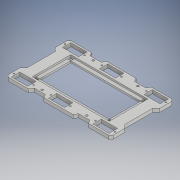
# Autodesk Inventor part: BODY_TOP
Saved by Autodesk Inventor 2017 (Build 210142000, 142)
## iProperties
Created: 2017-09-24
Part Number: BODY_TOP
Material: Generic
Document SubType Name: Modeling
Designer: Alexander Miller
Density: 1 g/cm^3
Appearance: Default
body_C_Top: 5,000 mm
Author: Alexander Miller
Autodesk Inventor part; units mm, degrees
ref_plane "YZ Plane" through (0, 0, 0) normal (1, 0, 0) x (0, 1, 0)
ref_plane "XZ Plane" through (0, 0, 0) normal (0, 1, 0) x (-1, 0, 0)
ref_plane "XY Plane" through (0, 0, 0) normal (0, 0, 1) x (1, 0, 0)
sketch "Sketch1" plane through (0, 0, 0) normal (0, 1, 0) x (-1, 0, 0)
  line L0 (45, -75) -> (-45, -75)
  line L1 (-45, -75) -> (-45, 75)
  line L2 (-45, 75) -> (45, 75)
  line L3 (45, 75) -> (45, -75)
  point P0 (0, 0)
  point P1 (0, -75)
  point P2 (45, 0)
  dimension "d0" = 90
  dimension "d1" = 150
  constraints: 8 end point, 2 midpoint, 2 parallel, 1 horizontal, 1 horizontal alignment, 1 perpendicular, 1 vertical alignment
  measures "d0" distance of L0.start L0.end
  measures "d1" distance of L2.end L0.start
extrude "Extrusion1" add sketch "Sketch1" along normal blind 5
sketch "Sketch2" plane through (0, 5, 0) normal (0, 1, 0) x (1, 0, 0)
  line L0 (-42.5, 69.75) -> (-30.5, 69.75)
  line L1 (-30.5, 69.75) -> (-30.5, 46.75)
  line L2 (-30.5, 46.75) -> (-42.5, 46.75)
  line L3 (-42.5, 46.75) -> (-42.5, 69.75)
  line L4 (-42.5, 17) -> (-30.5, 17)
  line L5 (-30.5, 17) -> (-30.5, -6)
  line L6 (-30.5, -6) -> (-42.5, -6)
  line L7 (-42.5, -6) -> (-42.5, 17)
  line L8 (-42.5, -46.75) -> (-30.5, -46.75)
  line L9 (-30.5, -46.75) -> (-30.5, -69.75)
  line L10 (-30.5, -69.75) -> (-42.5, -69.75)
  line L11 (-42.5, -69.75) -> (-42.5, -46.75)
  line L12 (-45, 75) -> (-45, -75) projected
  line L13 (45, 75) -> (-45, 75) projected
  line L14 (-45, -75) -> (45, -75) projected
  circle A0 centre (-36.5, 0) radius 6 construction
  circle A1 centre (-36.5, 72.25) radius 1
  circle A2 centre (-36.5, 44.25) radius 1
  circle A3 centre (-36.5, 19.5) radius 1
  circle A4 centre (-36.5, -8.5) radius 1
  circle A5 centre (-36.5, -44.25) radius 1
  circle A6 centre (-36.5, -72.25) radius 1
  line L15 (0, 105) -> (0, -105) construction
  line L16 (42.5, 69.75) -> (30.5, 69.75)
  line L17 (30.5, 69.75) -> (30.5, 46.75)
  line L18 (30.5, 46.75) -> (42.5, 46.75)
  line L19 (42.5, 46.75) -> (42.5, 69.75)
  line L20 (42.5, 17) -> (30.5, 17)
  line L21 (30.5, 17) -> (30.5, -6)
  line L22 (30.5, -6) -> (42.5, -6)
  line L23 (42.5, -6) -> (42.5, 17)
  line L24 (42.5, -46.75) -> (30.5, -46.75)
  line L25 (30.5, -46.75) -> (30.5, -69.75)
  line L26 (30.5, -69.75) -> (42.5, -69.75)
  line L27 (42.5, -69.75) -> (42.5, -46.75)
  circle A7 centre (36.5, 72.25) radius 1
  circle A8 centre (36.5, 44.25) radius 1
  circle A9 centre (36.5, 19.5) radius 1
  circle A10 centre (36.5, -8.5) radius 1
  circle A11 centre (36.5, -44.25) radius 1
  circle A12 centre (36.5, -72.25) radius 1
  point P0 (0, 0)
  point P1 (-36.5, 46.75)
  point P2 (-36.5, 17)
  point P3 (-36.5, -6)
  point P4 (-36.5, -46.75)
  point P5 (-36.5, 69.75)
  point P6 (-36.5, -69.75)
  dimension "d2" = 5
  dimension "d4" = 2.5
  dimension "d5" = 5.25
  dimension "d6" = 23
  dimension "d7" = 12
  dimension "d8" = 5.25
  dimension "d9" = 2
  dimension "d10" = 1.5
  dimension "d11" = 1.5
  dimension "d12" = 1.5
  dimension "d13" = 1.5
  dimension "d14" = 1.5
  dimension "d15" = 1.5
  constraints: 48 end point, 18 symmetric about line, 13 centre point, 8 vertical alignment, 6 midpoint, 6 parallel, 5 equal radius, 3 equal length, 3 horizontal, 3 perpendicular, 3 tangent, 2 point on line, 1 horizontal alignment, 6 other
  measures "d4" distance between parallel lines of L3 L12
  measures "d5" distance between parallel lines of L13 L0
  measures "d6" distance of L2.end L0.start
  measures "d7" distance of L0.start L0.end
  measures "d8" distance between parallel lines of L14 L10
  measures "d9" diameter of A1
  measures "d10" distance edge to line of A1 L0
  measures "d11" distance edge to line of A2 L2
  measures "d12" distance edge to line of A3 L4
  measures "d13" distance edge to line of A4 L6
  measures "d14" distance edge to line of A5 L8
  measures "d15" distance edge to line of A6 L10
extrude "Extrusion2" cut sketch "Sketch2" against normal through all
sketch "Sketch3" plane through (0, 5, 0) normal (0, 1, 0) x (1, 0, 0)
  line L0 (45, 42.875) -> (40, 39.875)
  line L1 (40, 39.875) -> (40, 23.875)
  line L2 (45, -75) -> (45, 75) projected
  line L3 (40, 23.875) -> (45, 20.875)
  line L4 (45, 20.875) -> (45, 42.875)
  line L5 (42.5, 46.75) -> (30.5, 46.75) projected
  line L6 (36.5, 46.75) -> (36.5, 17) construction
  line L7 (30.5, 17) -> (42.5, 17) projected
  line L8 (-63, 0) -> (63, 0) projected
  line L9 (0, 105) -> (0, -105) projected
  line L10 (45, -42.875) -> (40, -39.875)
  line L11 (40, -39.875) -> (40, -23.875)
  line L12 (40, -23.875) -> (45, -20.875)
  line L13 (45, -20.875) -> (45, -42.875)
  line L14 (-45, 42.875) -> (-40, 39.875)
  line L15 (-40, 39.875) -> (-40, 23.875)
  line L16 (-40, 23.875) -> (-45, 20.875)
  line L17 (-45, 20.875) -> (-45, 42.875)
  line L18 (-45, -42.875) -> (-40, -39.875)
  line L19 (-40, -39.875) -> (-40, -23.875)
  line L20 (-40, -23.875) -> (-45, -20.875)
  line L21 (-45, -20.875) -> (-45, -42.875)
  line L22 (25, 75) -> (-25, 75)
  line L23 (-25, 75) -> (-20, 70)
  line L24 (-20, 70) -> (20, 70)
  line L25 (20, 70) -> (25, 75)
  line L26 (45, 75) -> (-45, 75) projected
  line L27 (25, -75) -> (-25, -75)
  line L28 (-25, -75) -> (-20, -70)
  line L29 (-20, -70) -> (20, -70)
  line L30 (20, -70) -> (25, -75)
  point P0 (0, 0)
  point P1 (45, 31.875)
  point P2 (40, 31.875)
  point P3 (36.5, 31.875)
  point P4 (0, 70)
  point P5 (0, 75)
  dimension "d38" = 16
  dimension "d39" = 22
  dimension "d40" = 40
  dimension "d41" = 50
  dimension "d42" = 5
  dimension "d43" = 5
  constraints: 50 end point, 16 symmetric about line, 7 midpoint, 3 parallel, 2 collinear, 2 equal length, 2 horizontal alignment, 2 vertical alignment, 1 perpendicular
  measures "d38" distance of L0.end L1.end
  measures "d39" distance of L3.end L0.start
  measures "d40" distance of L23.end L24.end
  measures "d41" distance of L22.start L22.end
  measures "d42" distance between parallel lines of L26 L24
  measures "d43" distance between parallel lines of L1 L4
extrude "Extrusion3" cut sketch "Sketch3" against normal through all contours L2 L3 L1 L0 | L25 L24 L9 L22 | L9 L24 L23 L22 | L10 L11 L12 L2 | L29 L30 L27 L9 | L9 L27 L28 L29 | L14 L15 L16 L17 | L21 L20 L19 L18
chamfer "Chamfer1" distance 3 angle 45 4 edges at (45, 2.5, 75) (-45, 2.5, 75) (-45, 2.5, -75) (45, 2.5, -75)
sketch "Sketch4" plane through (0, 5, 0) normal (0, 1, 0) x (1, 0, 0)
  line L0 (27.5, 55) -> (-27.5, 55)
  line L1 (-27.5, 55) -> (-27.5, -55)
  line L2 (-27.5, -55) -> (27.5, -55)
  line L3 (27.5, -55) -> (27.5, 55)
  line L4 (22.5, 50) -> (-22.5, 50)
  line L5 (-22.5, 50) -> (-22.5, -50)
  line L6 (-22.5, -50) -> (22.5, -50)
  line L7 (22.5, -50) -> (22.5, 50)
  point P0 (0, 0)
  point P1 (27.5, 0)
  point P2 (0, 55)
  dimension "d23" = 110
  dimension "d24" = 55
  dimension "d25" = 5
  dimension "d26" = 5
  dimension "d27" = 5
  dimension "d28" = 5
  constraints: 16 end point, 4 parallel, 2 horizontal, 2 midpoint, 2 perpendicular, 1 horizontal alignment, 1 vertical alignment
  measures "d23" distance of L2.end L0.start
  measures "d24" distance of L1.end L2.end
  measures "d25" distance between parallel lines of L0 L4
  measures "d26" distance between parallel lines of L2 L6
  measures "d27" distance between parallel lines of L3 L7
  measures "d28" distance between parallel lines of L1 L5
extrude "Extrusion4" cut sketch "Sketch4" against normal blind 2.5
sketch "Sketch5" plane through (0, 5, 0) normal (0, 1, 0) x (1, 0, 0)
  line L0 (-22.5, 50) -> (-22.5, -50) projected
  line L1 (-22.5, -50) -> (22.5, -50) projected
  line L2 (22.5, -50) -> (22.5, 50) projected
  line L3 (22.5, 50) -> (-22.5, 50) projected
  point P0 (0, 0)
extrude "Extrusion5" cut sketch "Sketch5" against normal through all
sketch "Sketch6" plane through (0, 2.5, 0) normal (0, 1, 0) x (1, 0, 0)
  line L0 (27.5, 55) -> (22.5, 55)
  line L1 (22.5, 55) -> (22.5, 50)
  line L2 (22.5, 50) -> (27.5, 50)
  line L3 (27.5, 50) -> (27.5, 55)
  line L4 (-63, 0) -> (63, 0) projected
  line L5 (0, 105) -> (0, -105) projected
  line L6 (27.5, -55) -> (22.5, -55)
  line L7 (22.5, -55) -> (22.5, -50)
  line L8 (22.5, -50) -> (27.5, -50)
  line L9 (27.5, -50) -> (27.5, -55)
  line L10 (-27.5, 55) -> (-22.5, 55)
  line L11 (-22.5, 55) -> (-22.5, 50)
  line L12 (-22.5, 50) -> (-27.5, 50)
  line L13 (-27.5, 50) -> (-27.5, 55)
  line L14 (-27.5, -55) -> (-22.5, -55)
  line L15 (-22.5, -55) -> (-22.5, -50)
  line L16 (-22.5, -50) -> (-27.5, -50)
  line L17 (-27.5, -50) -> (-27.5, -55)
  line L18 (27.5, 55) -> (27.5, -55) projected
  line L19 (-27.5, 55) -> (27.5, 55) projected
  point P0 (0, 0)
  dimension "d33" = 5
  dimension "d34" = 5
  constraints: 32 end point, 12 symmetric about line, 2 collinear, 2 parallel, 1 horizontal, 1 perpendicular
  measures "d33" distance of L2.end L0.start
  measures "d34" distance of L1.end L2.end
extrude "Extrusion6" cut sketch "Sketch6" against normal blind 2 contours L3 L2 L1 L0 | L6 L7 L8 L9 | L10 L11 L12 L13 | L17 L16 L15 L14
sketch "Sketch7" plane through (0, 5, 0) normal (0, 1, 0) x (1, 0, 0)
  circle A0 centre (36.5, 31.875) radius 1.5
  line L0 (-63, 0) -> (63, 0) projected
  line L1 (0, 105) -> (0, -105) projected
  line L2 (40, 23.875) -> (40, 39.875) projected
  line L3 (30.5, 17) -> (42.5, 17) projected
  circle A1 centre (36.5, -31.875) radius 1.5
  circle A2 centre (-36.5, 31.875) radius 1.5
  circle A3 centre (-36.5, -31.875) radius 1.5
  point P0 (0, 0)
  point P1 (40, 31.875)
  point P2 (36.5, 17)
  dimension "d44" = 3
  constraints: 4 centre point, 3 symmetric about line, 2 midpoint, 1 horizontal alignment, 1 vertical alignment, 3 other
  measures "d44" diameter of A0
extrude "Extrusion7" cut sketch "Sketch7" against normal through all
sketch "Sketch8" plane through (0, 0, 0) normal (0, -1, 0) x (1, 0, 0)
  line L0 (-38.5, -46.25) -> (-34.5, -46.25)
  line L1 (-34.5, -46.25) -> (-34.5, -42.25)
  line L2 (-34.5, -42.25) -> (-38.5, -42.25)
  line L3 (-38.5, -42.25) -> (-38.5, -46.25)
  line L4 (-38.5, -74.25) -> (-34.5, -74.25)
  line L5 (-34.5, -74.25) -> (-34.5, -70.25)
  line L6 (-34.5, -70.25) -> (-38.5, -70.25)
  line L7 (-38.5, -70.25) -> (-38.5, -74.25)
  line L8 (-38.5, -21.5) -> (-34.5, -21.5)
  line L9 (-34.5, -21.5) -> (-34.5, -17.5)
  line L10 (-34.5, -17.5) -> (-38.5, -17.5)
  line L11 (-38.5, -17.5) -> (-38.5, -21.5)
  line L12 (-38.5, 6.5) -> (-34.5, 6.5)
  line L13 (-34.5, 6.5) -> (-34.5, 10.5)
  line L14 (-34.5, 10.5) -> (-38.5, 10.5)
  line L15 (-38.5, 10.5) -> (-38.5, 6.5)
  line L16 (-38.5, 42.25) -> (-34.5, 42.25)
  line L17 (-34.5, 42.25) -> (-34.5, 46.25)
  line L18 (-34.5, 46.25) -> (-38.5, 46.25)
  line L19 (-38.5, 46.25) -> (-38.5, 42.25)
  line L20 (-34.5, 70.25) -> (-38.5, 70.25)
  line L21 (-38.5, 70.25) -> (-38.5, 74.25)
  line L22 (-38.5, 74.25) -> (-34.5, 74.25)
  line L23 (-34.5, 74.25) -> (-34.5, 70.25)
  circle A0 centre (-36.5, -72.25) radius 1 projected
  circle A1 centre (-36.5, -44.25) radius 1 projected
  circle A2 centre (-36.5, -19.5) radius 1 projected
  circle A3 centre (-36.5, 8.5) radius 1 projected
  circle A4 centre (-36.5, 44.25) radius 1 projected
  circle A5 centre (-36.5, 72.25) radius 1 projected
  line L24 (0, -105.35) -> (0, 105.35) projected
  line L25 (38.5, -46.25) -> (34.5, -46.25)
  line L26 (34.5, -46.25) -> (34.5, -42.25)
  line L27 (34.5, -42.25) -> (38.5, -42.25)
  line L28 (38.5, -42.25) -> (38.5, -46.25)
  line L29 (38.5, -74.25) -> (34.5, -74.25)
  line L30 (34.5, -74.25) -> (34.5, -70.25)
  line L31 (34.5, -70.25) -> (38.5, -70.25)
  line L32 (38.5, -70.25) -> (38.5, -74.25)
  line L33 (38.5, -21.5) -> (34.5, -21.5)
  line L34 (34.5, -21.5) -> (34.5, -17.5)
  line L35 (34.5, -17.5) -> (38.5, -17.5)
  line L36 (38.5, -17.5) -> (38.5, -21.5)
  line L37 (38.5, 6.5) -> (34.5, 6.5)
  line L38 (34.5, 6.5) -> (34.5, 10.5)
  line L39 (34.5, 10.5) -> (38.5, 10.5)
  line L40 (38.5, 10.5) -> (38.5, 6.5)
  line L41 (38.5, 42.25) -> (34.5, 42.25)
  line L42 (34.5, 42.25) -> (34.5, 46.25)
  line L43 (34.5, 46.25) -> (38.5, 46.25)
  line L44 (38.5, 46.25) -> (38.5, 42.25)
  line L45 (34.5, 70.25) -> (38.5, 70.25)
  line L46 (38.5, 70.25) -> (38.5, 74.25)
  line L47 (38.5, 74.25) -> (34.5, 74.25)
  line L48 (34.5, 74.25) -> (34.5, 70.25)
  point P0 (0, 0)
  point P1 (-36.5, -74.25)
  point P2 (-36.5, -46.25)
  point P3 (-36.5, -42.25)
  point P4 (-36.5, -21.5)
  point P5 (-36.5, -17.5)
  point P6 (-36.5, 6.5)
  point P7 (-36.5, 10.5)
  point P8 (-36.5, 42.25)
  point P9 (-36.5, 46.25)
  point P10 (-36.5, 70.25)
  point P11 (-38.5, -72.25)
  point P12 (-38.5, -44.25)
  point P13 (-38.5, -19.5)
  point P14 (-38.5, 8.5)
  point P15 (-38.5, 72.25)
  point P16 (-38.5, 44.25)
  dimension "d47" = 4
  constraints: 96 end point, 24 symmetric about line, 16 midpoint, 12 parallel, 11 equal length, 6 horizontal, 6 horizontal alignment, 6 perpendicular, 6 vertical alignment, 2 point on line
  measures "d47" distance of L6.end L4.start
extrude "Extrusion8" cut sketch "Sketch8" against normal blind 1.2
equation "\"d0\" = body_B"
equation "\"d1\" = body_A"
equation "\"d2\" = body_C_Top"
equation "\"d4\" = 0.5 * body_C"
equation "\"d6\" = servo_A"
equation "\"d7\" = servo_B"
equation "\"d8\" = d5"
equation "\"d9\" = servo_H"
equation "\"d10\" = servo_L"
equation "\"d11\" = d10"
equation "\"d12\" = d10"
equation "\"d13\" = d10"
equation "\"d14\" = d10"
equation "\"d15\" = d10"
equation "\"d16\" = body_C"
equation "\"d26\" = d25"
equation "\"d27\" = d25"
equation "\"d28\" = d25"
equation "\"d29\" = 0.5 * body_C"
equation "\"d31\" = 0.5 * body_C"
equation "\"d33\" = magnet_A"
equation "\"d34\" = magnet_A"
equation "\"d35\" = magnet_B"
equation "\"d44\" = nut_C"
equation "\"d47\" = nut_A_1"
equation "\"d48\" = nut_B_1"
equation "\"body_C_Top\" = body_C"
equation "\"body_B\" = 90"
equation "\"body_A\" = 150"
equation "\"body_C\" = 5"
equation "\"servo_A\" = 23"
equation "\"servo_B\" = 12"
equation "\"servo_H\" = 2"
equation "\"servo_L\" = 1.5"
equation "\"magnet_A\" = 5"
equation "\"magnet_B\" = 2"
equation "\"nut_C\" = 3"
equation "\"nut_A_1\" = 4"
equation "\"nut_B_1\" = 1.2"
body "Solid1"
